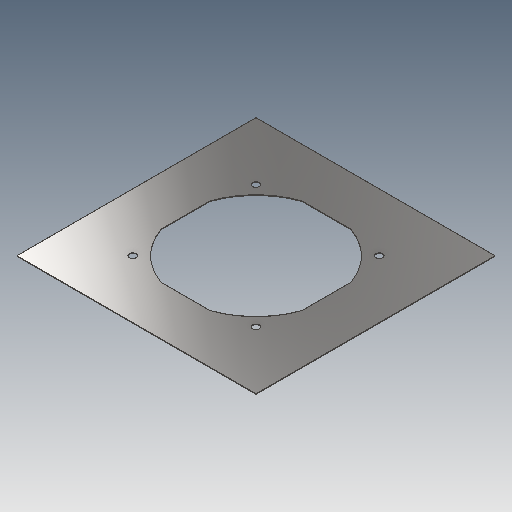
# Autodesk Inventor part: top panel
Saved by Autodesk Inventor 2027 (Build 310192060, 192F)
## iProperties
Created: 2026-07-27
Part Number: top panel
Material: Stainless Steel
Document SubType Name: Sheet Metal
Designer: prest
Density: 8 g/cm^3
Sheet Metal Rule: Default_mm
Appearance: Semi-Polished
Author: prest
Autodesk Inventor part; units mm, degrees
ref_plane "YZ Plane" through (0, 0, 0) normal (1, 0, 0) x (0, 1, 0)
ref_plane "XZ Plane" through (0, 0, 0) normal (0, 1, 0) x (-1, 0, 0)
ref_plane "XY Plane" through (0, 0, 0) normal (0, 0, 1) x (1, 0, 0)
sketch "Sketch1" plane through (0, 0, 0) normal (0, 1, 0) x (-1, 0, 0)
  line L0 (101.8, 101.8) -> (-101.8, 101.8)
  line L1 (-101.8, 101.8) -> (-101.8, -101.8)
  line L2 (-101.8, -101.8) -> (101.8, -101.8)
  line L3 (101.8, -101.8) -> (101.8, 101.8)
  point P0 (0, 101.8)
  point P1 (101.8, 0)
  dimension "d0" = 203.6
  dimension "d1" = 203.6
  measures "d0" distance of L0.start L0.end
  measures "d1" distance of L0.end L1.end
extrude "Plate1" add sketch "Sketch1" along normal blind 0.5
sketch "Sketch2" plane through (0, 0.5, 0) normal (0, 1, 0) x (1, 0, 0)
  line L0 (-52.5, -52.5) -> (52.5, 52.5) construction
  line L1 (52.5, -52.5) -> (-52.5, 52.5) construction
  point P0 (0, 0)
  point P1 (0, 0)
  dimension "d7" = 105
  dimension "d8" = 105
  constraints: 4 end point, 2 horizontal alignment, 2 vertical alignment, 1 coincident, 1 midpoint
  measures "d7" distance of L1.start L0.start
  measures "d8" distance of L1.end L0.start
hole "Hole1" at (-52.5, 0.5, 52.5) at (-52.5, 0.5, -52.5) at (52.5, 0.5, 52.5) at (52.5, 0.5, -52.5) direction (0, -1, 0) diameter 6 depth 0.5 tip angle 118
sketch "Sketch3" plane through (0, 0.5, 0) normal (0, 1, 0) x (1, 0, 0)
  line L0 (-60, -60) -> (60, -60)
  line L1 (60, -60) -> (60, 60)
  line L2 (60, 60) -> (-60, 60)
  line L3 (-60, 60) -> (-60, -60)
  arc A0 (-60, -20.7906) -> (-20.7906, -60) centre (0, 0) ccw
  arc A1 (20.7906, -60) -> (60, -20.7906) centre (0, 0) ccw
  arc A2 (60, 20.7906) -> (20.7906, 60) centre (0, 0) ccw
  arc A3 (-20.7906, 60) -> (-60, 20.7906) centre (0, 0) ccw
  point P0 (0, -48.7613)
  point P1 (-70.0637, 0)
  point P2 (-60, 0)
  point P3 (0, -60)
  dimension "d17" = 120
  constraints: 8 end point, 8 point on circle, 8 point on line, 4 centre point, 2 horizontal alignment, 2 midpoint, 2 parallel, 2 perpendicular, 2 vertical alignment, 1 coincident, 1 horizontal
  measures "d17" distance of L0.start L0.end
extrude "Cut1" cut sketch "Sketch3" against normal blind 0.5 contours A0 L3 A3 L2 A2 L1 A1 L0
equation "\"d8\" = d7"
equation "\"d14\" = Thickness"
equation "\"d19\" = Thickness"
equation "\"d2\" = Thickness"
equation "\"BendRadius\" = Thickness"
equation "\"BendReliefWidth\" = Thickness"
equation "\"BendReliefDepth\" = 0.5 * Thickness"
equation "\"CornerReliefSize\" = 4 * Thickness"
equation "\"MinimumRemnant\" = 2 * Thickness"
equation "\"TransitionRadius\" = BendRadius"
equation "\"JacobiRadiusSize\" = BendRadius"
equation "\"GapSize\" = Thickness"
equation "\"Thickness\" = 0.5"
body "Solid1"
